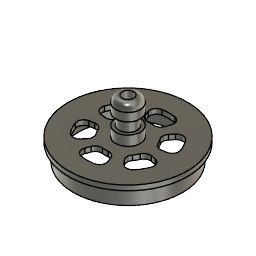
Back Reel Shaft (Autodesk Fusion 360 design; units mm, degrees)
Autodesk Fusion 360 part; units mm, degrees
sketch "Sketch1" plane through (0, 0, 0) normal (0, 0, 1) x (1, 0, 0)
  circle A0 centre (0, 0) radius 30.4
  circle A1 centre (0, 0) radius 33.4
  circle A2 centre (0, 0) radius 36.4
  circle A3 centre (0, 0) radius 7.5
  circle A4 centre (0, 0) radius 14
  line L0 (0, 0) -> (4.7883, -13.1557)
  line L1 (0, 0) -> (-4.7883, -13.1557)
  line L2 (0, -60) -> (0, 60)
  line L3 (4.7883, -13.1557) -> (8.5505, -23.4923)
  line L4 (-4.7883, -13.1557) -> (-8.5505, -23.4923)
  arc A5 (8.5505, -23.4923) -> (-8.5505, -23.4923) centre (0, 0) ccw
  arc A6 (-8.5505, -23.4923) -> (0, -25) centre (0, 0) ccw
  arc A7 (0, -25) -> (8.5505, -23.4923) centre (0, 0) ccw
  line L5 (13.7873, -2.4311) -> (24.6202, -4.3412)
  line L6 (8.999, -10.7246) -> (16.0697, -19.1511)
  line L7 (8.999, 10.7246) -> (16.0697, 19.1511)
  line L8 (13.7873, 2.4311) -> (24.6202, 4.3412)
  line L9 (-4.7883, 13.1557) -> (-8.5505, 23.4923)
  line L10 (4.7883, 13.1557) -> (8.5505, 23.4923)
  line L11 (-13.7873, 2.4311) -> (-24.6202, 4.3412)
  line L12 (-8.999, 10.7246) -> (-16.0697, 19.1511)
  line L13 (-8.999, -10.7246) -> (-16.0697, -19.1511)
  line L14 (-13.7873, -2.4311) -> (-24.6202, -4.3412)
  circle A8 centre (0, 0) radius 3.5
  circle A9 centre (0, 0) radius 5.5
  point P0 (0, 7.5)
  dimension "d1" = 60.8
  dimension "d2" = 3
  dimension "d3" = 3
  dimension "d4" = 15
  dimension "d11" = 28
  dimension "d12" = 50
  dimension "d13" = 40
  dimension "d15" = 20
  dimension "d17" = 360
  dimension "d22" = -4
  dimension "d34" = -2
  constraint coincident A0.centre A1.centre
  constraint concentric A0 A3
  constraint concentric A0 A5
  constraint concentric A0 A4
  constraint vertical L2
  constraint coincident A4 L0.end
  constraint coincident A4 L1.end
  constraint coincident L2 A6.end
  constraint concentric A5 A6
  constraint concentric A5 A7
  constraint coincident A3 P0
  constraint coincident L2 P0
  constraint coincident A0.centre L2
  measures "d1" diameter of A0
  measures "d4" diameter of A3
  measures "d11" diameter of A4
  measures "d12" diameter of A5
  measures "d13" angle of L0 L1
  measures "d15" angle of L1 L2
extrude "Extrude1" add sketch "Sketch1" against normal blind 10 contours A0 A1 L2 | A0 A1 L2
extrude "Extrude2" add sketch "Sketch1" along normal blind 3
extrude "Extrude3" add sketch "Sketch1" along normal blind 25 contours A3 L1 L2 A9 | A3 L0 L2 A9 | A3 L0 L2 A9 | A3 L1 L2 A9 | L0 L2 A8 A9 | L1 L2 A8 A9 | L1 L2 A8 A9 | L0 L2 A8 A9 | L0 L2 A8 | L1 L2 A8 | L1 L2 A8 | L0 L2 A8
extrude "Extrude4" cut sketch "Sketch1" along normal blind 3 contours A4 L2 A5 L10 | A4 L2 A5 L9 | A4 L2 L4 A6 | A4 L2 L3 A7 | A4 A5 L7 L8 | A4 A5 L11 L12 | A4 A5 L13 L14 | A4 A5 L5 L6
fillet "Fillet1" radius 4 24 edges at (-16.0697, 19.1511, 1.5) (-24.6202, 4.3412, 1.5) (-13.7873, 2.4311, 1.5) (-8.999, 10.7246, 1.5) (-13.7873, -2.4311, 1.5) (-24.6202, -4.3412, 1.5) (-16.0697, -19.1511, 1.5) (-8.999, -10.7246, 1.5) (-4.7883, -13.1557, 1.5) (-8.5505, -23.4923, 1.5) (8.5505, -23.4923, 1.5) (4.7883, -13.1557, 1.5) (8.999, -10.7246, 1.5) (16.0697, -19.1511, 1.5) (24.6202, -4.3412, 1.5) (13.7873, -2.4311, 1.5) (24.6202, 4.3412, 1.5) (16.0697, 19.1511, 1.5) (13.7873, 2.4311, 1.5) (8.999, 10.7246, 1.5) (4.7883, 13.1557, 1.5) (8.5505, 23.4923, 1.5) (-4.7883, 13.1557, 1.5) (-8.5505, 23.4923, 1.5)
extrude "Extrude5" cut sketch "Sketch1" against normal up to surface (22 mm away) from surface at 25 contours L0 L2 A8 | L1 L2 A8 | L1 L2 A8 | L0 L2 A8
extrude "Extrude7" cut sketch "Sketch1" along normal blind 7 from surface at 9 contours A3 L1 L2 A9 | A3 L0 L2 A9 | A3 L0 L2 A9 | A3 L1 L2 A9
fillet "Fillet4" radius 4 1 edges at (-6.9925, -2.7121, 25)
